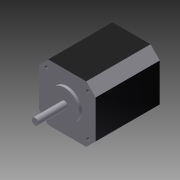
# Autodesk Inventor part: SM-E01
Saved by Autodesk Inventor 2014 (Build 180170000, 170)
## iProperties
Created: 2011-08-01
Part Number: SM-E01
Document SubType Name: Modeling
Designer: ERF
Density: 4.31853 g/cm^3
Description: Stepper Motor - NEMA17 60oz/in 200steps / rev
Vendor: automation technology
Mass: 358.338 g
Surface Area: 115.445 cm^2
Volume: 82.9768 cm^3
Material: Aluminum-6061
Stock Number: B10-10001
Project: Shapeoko
Appearance: Aluminum - Flat
Author: ERF
Title: Nema 17 Stepper Motor (60oz/in holding torque)
Autodesk Inventor part; units mm, degrees
ref_plane "YZ Plane" through (0, 0, 0) normal (1, 0, 0) x (0, 1, 0)
ref_plane "XZ Plane" through (0, 0, 0) normal (0, 1, 0) x (-1, 0, 0)
ref_plane "XY Plane" through (0, 0, 0) normal (0, 0, 1) x (1, 0, 0)
sketch "Sketch1" plane through (0, 0, 0) normal (0, 0, 1) x (1, 0, 0)
  line L0 (20.2828, 57.747) -> (62.7008, 57.747)
  line L1 (62.7008, 57.747) -> (62.7008, 15.329)
  line L2 (62.7008, 15.329) -> (20.2828, 15.329)
  line L3 (20.2828, 15.329) -> (20.2828, 57.747)
  dimension "d0" = 42.418
  dimension "d1" = 42.418
  constraints: 8 end point, 2 parallel, 1 horizontal, 1 perpendicular
  measures "d0" distance of L0.start L0.end
  measures "d1" distance between parallel lines of L0 L2
extrude "Extrusion1" add sketch "Sketch1" along normal blind 48.006
sketch "Sketch2" plane through (0, 0, 48.006) normal (0, 0, 1) x (1, 0, 0)
  line L0 (20.2828, 57.747) -> (62.7008, 57.747) projected
  line L1 (20.2828, 15.329) -> (20.2828, 57.747) projected
  circle A0 centre (25.9978, 52.032) radius 1.5
  dimension "d4" = 3
  dimension "d5" = 5.715
  dimension "d6" = 5.715
  constraints: 1 centre point
  measures "d4" diameter of A0
  measures "d5" distance from line of L1 A0.centre
  measures "d6" distance from line of L0 A0.centre
hole "Hole1" at (25.9978, 52.032, 48.006) direction (0, 0, -1) diameter 2.4638 depth 4.5 tip angle 118
pattern_linear "Rectangular Pattern1" count 2 spacing 31 along (1, 0, 0) count 2 spacing 31 along (0, -1, 0) of "Hole1"
sketch "Sketch3" plane through (0, 0, 48.006) normal (0, 0, 1) x (1, 0, 0)
  circle A0 centre (41.4918, 36.538) radius 11.049
  dimension "d20" = 22.098
  constraints: 1 centre point
  measures "d20" diameter of A0
extrude "Extrusion2" add sketch "Sketch3" along normal blind 2
sketch "Sketch4" plane through (41.4918, 36.538, 50.006) normal (0, 0, 1) x (1, 0, 0)
  circle A0 centre (0, 0) radius 11.049 projected
  circle A1 centre (0, 0) radius 2.5
  dimension "d23" = 5
  constraints: 1 centre point, 1 coincident
  measures "d23" diameter of A1
extrude "Extrusion3" add sketch "Sketch4" along normal blind 22 contours A1
chamfer "Chamfer1" distance 7 angle 45 4 edges at (62.7008, 57.747, 24.003) (20.2828, 57.747, 24.003) (20.2828, 15.329, 24.003) (62.7008, 15.329, 24.003)
sketch "Sketch5" plane through (0, 0, 0) normal (0, 0, -1) x (-1, 0, 0)
  line L0 (-27.2828, 57.747) -> (-55.7008, 57.747) projected
  line L1 (-62.7008, 50.747) -> (-62.7008, 22.329) projected
  circle A0 centre (-41.4918, 36.538) radius 2.5
  dimension "d29" = 5
  dimension "d30" = 21.209
  dimension "d31" = 21.209
  constraints: 1 centre point
  measures "d29" diameter of A0
  measures "d30" distance from line of L0 A0.centre
  measures "d31" distance from line of L1 A0.centre
extrude "Extrusion4" add sketch "Sketch5" along normal blind 10
body "Solid1"
